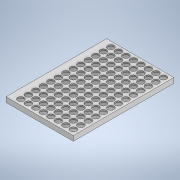
# Autodesk Inventor part: WasherTrayForRobot
Saved by Autodesk Inventor 2020 (Build 240168000, 168)
## iProperties
Created: 2021-07-14
Part Number: WasherTrayForRobot
Material: Generic
Document SubType Name: Modeling
Designer: pab2
Density: 1 g/cm^3
Appearance: Default
Author: pab2
Autodesk Inventor part; units mm, degrees
ref_plane "YZ Plane" through (0, 0, 0) normal (1, 0, 0) x (0, 1, 0)
ref_plane "XZ Plane" through (0, 0, 0) normal (0, 1, 0) x (-1, 0, 0)
ref_plane "XY Plane" through (0, 0, 0) normal (0, 0, 1) x (1, 0, 0)
sketch "Sketch1" plane through (0, 0, 0) normal (0, 1, 0) x (-1, 0, 0)
  line L0 (0, 0) -> (85.48, 0)
  line L1 (85.48, 0) -> (85.48, -127.76)
  line L2 (85.48, -127.76) -> (0, -127.76)
  line L3 (0, -127.76) -> (0, 0)
  line L4 (0, 0) -> (7.0711, -7.0711)
  line L5 (0, 0) -> (10, 0) construction
  circle A0 centre (7.0711, -7.0711) radius 4.7625
  dimension "d0" = 85.48
  dimension "d1" = 127.76
  dimension "offsetDiag" = 10
  dimension "d3" = 45
  dimension "d4" = 9.525
  constraints: 12 end point, 2 horizontal, 2 parallel, 1 centre point, 1 coincident, 1 equal length, 1 perpendicular
  measures "d0" distance of L1.end L2.end
  measures "d1" distance of L0.end L1.end
  measures "offsetDiag" distance of L0.start L4.end
  measures "d3" angle of L4 L5
  measures "d4" diameter of A0
extrude "Extrusion1" add sketch "Sketch1" along normal blind 6.35 contours L0 L1 L2 L3 | A0
sketch "Sketch2" plane through (0, 6.35, 0) normal (0, 1, 0) x (1, 0, 0)
  line L0 (-85.48, 0) -> (0, 0) projected
  line L1 (0, 0) -> (-6.7352, 6.7352)
  line L2 (0, 0) -> (9.525, 0) construction
  circle A0 centre (-6.7352, 6.7352) radius 4.7625
  dimension "d7" = 9.525
  dimension "d8" = 135
  dimension "d9" = 9.525
  constraints: 4 end point, 1 centre point, 1 coincident, 1 equal length, 1 horizontal
  measures "d7" distance of L0.end L1.end
  measures "d8" angle of L2 L1
  measures "d9" diameter of A0
hole "Hole1" at (-6.7352, 6.35, -6.7352) direction (0, -1, 0) diameter 7.9375 depth 1.5875 tip angle 118
pattern_linear "Rectangular Pattern1" count 8 spacing 9.525 along (-1, 0, 0) count 13 spacing 9.525 along (0, 0, -1) of "Hole1"
body "Solid1"
